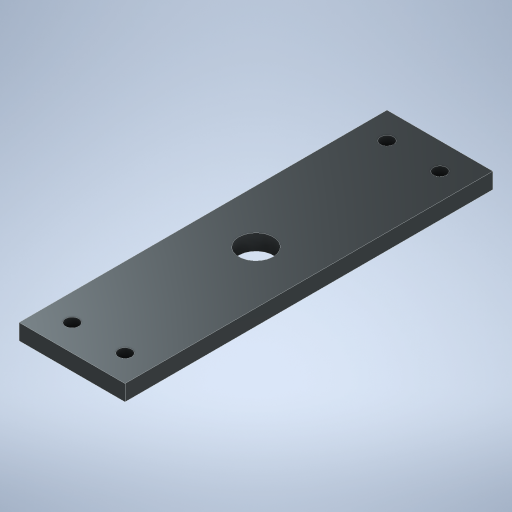
# Autodesk Inventor part: Contra ponto
Saved by Autodesk Inventor 2023.2 (Build 272271030, 271C)
## iProperties
Created: 2023-03-21
Part Number: Contra ponto
Material: Aço
Document SubType Name: Sheet Metal
Designer: Mateus
Density: 7.85 g/cm^3
Sheet Metal Rule: Padrão_mm
Appearance: Ferro cinza
Mass: 202.706 g
Surface Area: 111.975 cm^2
Volume: 25.8224 cm^3
Author: Mateus
Autodesk Inventor part; units mm, degrees
ref_plane "YZ Plane" through (0, 0, 0) normal (1, 0, 0) x (0, 1, 0)
ref_plane "XZ Plane" through (0, 0, 0) normal (0, 1, 0) x (-1, 0, 0)
ref_plane "XY Plane" through (0, 0, 0) normal (0, 0, 1) x (1, 0, 0)
sketch "Esboço1" plane through (0, 0, 0) normal (0, 1, 0) x (-1, 0, 0)
  line L0 (0, 0) -> (40, 0)
  line L1 (40, 0) -> (40, -139)
  line L2 (40, -139) -> (0, -139)
  line L3 (0, -139) -> (0, 0)
  dimension "d0" = 40
  dimension "d1" = 139
  constraints: 8 end point, 2 parallel, 1 horizontal, 1 perpendicular
  measures "d0" distance of L1.end L2.end
  measures "d1" distance of L0.end L1.end
extrude "Extrusão1" add sketch "Esboço1" along normal blind 6
sketch "Esboço2" plane through (0, 6, 0) normal (0, 1, 0) x (1, 0, 0)
  line L0 (-40, 139) -> (-40, 0) projected
  line L1 (-40, 0) -> (0, 0) projected
  point P0 (-20, 69.5)
  dimension "d4" = 139
  dimension "d5" = 40
  dimension "d6" = 20
  dimension "d7" = 69.5
  measures "d4" distance of L0.start L0.end
  measures "d5" distance of L0.end L1.end
  measures "d6" distance from line of L0 point (-20, 69.5)
  measures "d7" distance from line of L1 point (-20, 69.5)
hole "Furo1" at (-20, 6, -69.5) direction (0, -1, 0) diameter 13 depth 6 tip angle 118
sketch "Esboço3" plane through (0, 6, 0) normal (0, 1, 0) x (1, 0, 0)
  line L0 (0, 139) -> (-40, 139) projected
  line L1 (-40, 0) -> (0, 0) projected
  line L2 (-40, 139) -> (-40, 0) projected
  line L3 (0, 0) -> (0, 139) projected
  point P0 (-4.5, 4.5)
  point P1 (-35.5, 4.5)
  point P2 (-4.5, 134.5)
  point P3 (-35.5, 134.5)
  point P4 (-35.5, 103.5)
  point P5 (-4.5, 103.5)
  point P6 (-4.5, 4.5)
  point P7 (-4.5, 35.5)
  point P8 (-35.5, 35.5)
  dimension "d19" = 40
  dimension "d22" = 4.5
  dimension "d23" = 4.5
  dimension "d32" = 0
  dimension "d33" = 4.5
  dimension "d34" = 0
  dimension "d35" = 31
  dimension "d36" = 31
  dimension "d37" = 31
  dimension "d38" = 31
  dimension "d39" = 31
  dimension "d40" = 31
  dimension "d41" = 31
  dimension "d42" = 4.5
  dimension "d43" = 0
  dimension "d44" = 4.5
  constraints: 1 coincident
  measures "d19" distance of L1.start L1.end
  measures "d22" distance from line of L3 point (-4.5, 134.5)
  measures "d23" distance from line of L2 point (-35.5, 134.5)
  measures "d32" vertical distance of point (-4.5, 134.5) point (-35.5, 134.5)
  measures "d33" distance from line of L1 point (-4.5, 4.5)
  measures "d34" vertical distance of point (-35.5, 4.5) point (-4.5, 4.5)
  measures "d35" distance of point (-35.5, 4.5) point (-4.5, 4.5)
  measures "d36" distance of point (-4.5, 4.5) point (-4.5, 35.5)
  measures "d37" distance of point (-35.5, 4.5) point (-35.5, 35.5)
  measures "d38" distance of point (-4.5, 35.5) point (-35.5, 35.5)
  measures "d39" distance of point (-35.5, 134.5) point (-35.5, 103.5)
  measures "d40" distance of point (-4.5, 103.5) point (-4.5, 134.5)
  measures "d41" distance of point (-35.5, 103.5) point (-4.5, 103.5)
  measures "d42" distance from line of L0 point (-4.5, 134.5)
  measures "d43" horizontal distance of point (-35.5, 4.5) point (-35.5, 35.5)
  measures "d44" distance from line of L2 point (-35.5, 35.5)
hole "Furo2" [suppressed]
sketch "Esboço4" plane through (0, 6, 0) normal (0, 1, 0) x (1, 0, 0)
  line L0 (0, 139) -> (-40, 139) projected
  line L1 (0, 0) -> (0, 139) projected
  line L2 (-40, 0) -> (0, 0) projected
  line L3 (-40, 139) -> (-40, 0) projected
  point P0 (-10, 10)
  point P1 (-10, 129)
  point P2 (-20, 0)
  point P3 (-30, 129)
  point P4 (-30, 10)
  dimension "d45" = 40
  dimension "d46" = 10
  dimension "d47" = 10
  dimension "d48" = 10
  dimension "d49" = 10
  dimension "d57" = 10
  dimension "d58" = 10
  dimension "d59" = 10
  constraints: 1 midpoint
  measures "d45" distance of L0.start L0.end
  measures "d46" distance from line of L1 point (-10, 129)
  measures "d47" distance from line of L0 point (-10, 129)
  measures "d48" horizontal distance of point (-20, 0) point (-10, 10)
  measures "d49" distance from line of L1 point (-10, 10)
  measures "d57" distance from line of L3 point (-30, 10)
  measures "d58" distance from line of point (-30, 129) L3
  measures "d59" distance from line of L0 point (-30, 129)
hole "Furo3" at (-10, 6, -10) at (-10, 6, -129) at (-30, 6, -10) at (-30, 6, -129) direction (0, -1, 0) diameter 5 end through all
equation "\"d6\" = 0.5 * d5"
equation "\"d7\" = 0.5 * d4"
equation "\"d13\" = Espessura"
equation "\"d42\" = d23"
equation "\"d48\" = d47"
equation "\"d57\" = d49"
equation "\"d58\" = d46"
equation "\"d59\" = d47"
equation "\"d29\" = Espessura"
equation "\"d55\" = Espessura"
equation "\"Raio_vergadura\" = Espessura"
equation "\"Largura_alívio_de_vergadura\" = Espessura"
equation "\"Profundidade_alívio_de_vergadura\" = 0.5 * Espessura"
equation "\"Tamanho_alívio_de_dobra\" = 4 * Espessura"
equation "\"Remanescente_mínimo\" = 2 * Espessura"
equation "\"Raiodetransição\" = Raio_vergadura"
equation "\"Tamanho_de_raio_de_Jacobi\" = Raio_vergadura"
equation "\"TamanhoFolga\" = Espessura"
equation "\"Espessura\" = 0.5"
